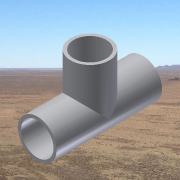
# Autodesk Inventor part: 0pvc_T_0.75
Saved by Autodesk Inventor 2014 SP1 (Build 180222100, 222)
## iProperties
Company: HERA Project
Created: 2013-06-12
Part Number: 0pvc_T_0.75
Material: PVC-Piping
Document SubType Name: Modeling
Designer: David DeBoer
Density: 1.4 g/cm^3
Description: 3/4" PVC Tee
Mass: 47.0427 g
Surface Area: 211.064 cm^2
Volume: 33.6019 cm^3
Appearance: Smooth - White
Author: David DeBoer
Title: PVC-T-0.75
Autodesk Inventor part; units mm, degrees
ref_plane "YZ Plane" through (0, 0, 0) normal (1, 0, 0) x (0, 1, 0)
ref_plane "XZ Plane" through (0, 0, 0) normal (0, 1, 0) x (-1, 0, 0)
ref_plane "XY Plane" through (0, 0, 0) normal (0, 0, 1) x (1, 0, 0)
sketch "Sketch1" plane through (0, 0, 0) normal (0, 0, 1) x (1, 0, 0)
  circle A0 centre (0, 0) radius 15.875
  dimension "d0" = 31.75
  constraints: 1 centre point, 1 coincident
  measures "d0" diameter of A0
extrude "mainBody" add sketch "Sketch1" along normal blind 86.5188
sketch "Sketch10" plane through (0, 0, 86.5188) normal (0, 0, 1) x (1, 0, 0)
  circle A0 centre (0, 0) radius 30.1625 projected
  circle A1 centre (0, 0) radius 15.875 projected
  point P0 (0, 15.875)
  constraints: 1 vertical alignment, 1 other
ref_plane "Work Plane5" through (0, 15.875, 86.5188) normal (0, 1, 0) x (-1, 0, 0)
sketch "Sketch11" plane through (0, 15.875, 86.5188) normal (0, 1, 0) x (-1, 0, 0)
  circle A0 centre (0, -43.2594) radius 15.875
  line L0 (15.875, 0) -> (-15.875, 0) projected
  point P0 (0, -86.5188)
  dimension "d29" = 43.2594
  dimension "d30" = 31.75
  constraints: 1 centre point
  measures "d29" distance from line of A0.centre L0
  measures "d30" diameter of A0
extrude "TBody" add sketch "Sketch11" along normal blind 26.1938 and the other way blind 16.51
sketch "Sketch12" plane through (0, 42.0688, 43.2594) normal (0, 1, 0) x (1, 0, 0)
  circle A0 centre (0, 0) radius 15.875 projected
  circle A1 centre (0, 0) radius 13.335
  point P0 (0, 43.2594)
  dimension "d35" = 26.67
  constraints: 1 centre point, 1 coincident
  measures "d35" diameter of A1
extrude "TSocket" cut sketch "Sketch12" against normal blind 25.4 contours A1
sketch "Sketch13" plane through (0, 16.6688, 43.2594) normal (0, 1, 0) x (1, 0, 0)
  circle A0 centre (0, 0) radius 13.335 projected
  circle A1 centre (0, 0) radius 10.4648
  point P0 (0, 43.2594)
  dimension "d39" = 20.9296
  constraints: 1 centre point, 1 coincident
  measures "d39" diameter of A1
extrude "TTube" cut sketch "Sketch13" against normal blind 15.24 contours A1
sketch "Sketch14" plane through (0, 0, 86.5188) normal (0, 0, 1) x (1, 0, 0)
  circle A0 centre (0, 0) radius 15.875 projected
  circle A1 centre (0, 0) radius 10.4648
  dimension "d43" = 20.9296
  constraints: 1 centre point, 1 coincident
  measures "d43" diameter of A1
extrude "mainTube" cut sketch "Sketch14" against normal blind 177.8 contours A1
sketch "Sketch15" plane through (0, 0, 86.5188) normal (0, 0, 1) x (1, 0, 0)
  circle A0 centre (0, 0) radius 10.4648 projected
  circle A1 centre (0, 0) radius 15.875 projected
  circle A2 centre (0, 0) radius 13.335
  dimension "d47" = 26.67
  constraints: 1 centre point, 1 coincident
  measures "d47" diameter of A2
extrude "mainSocket1" cut sketch "Sketch15" against normal blind 25.4 contours A2
sketch "Sketch16" plane through (0, 0, 0) normal (0, 0, -1) x (-1, 0, 0)
  circle A0 centre (0, 0) radius 10.4648 projected
  circle A1 centre (0, 0) radius 15.875 projected
  circle A2 centre (0, 0) radius 13.335
  dimension "d51" = 26.67
  constraints: 1 centre point, 1 coincident
  measures "d51" diameter of A2
extrude "mainSocket2" cut sketch "Sketch16" against normal blind 25.4 contours A2
body "Solid1"
